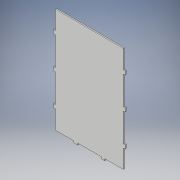
# Autodesk Inventor part: BB Gun Floor
Saved by Autodesk Inventor 2018 (Build 220112000, 112)
## iProperties
Created: 2019-05-24
Part Number: BB Gun Floor
Material: Generic
Document SubType Name: Modeling
Designer: 871357
Density: 1 g/cm^3
Appearance: Default
Author: 871357
Autodesk Inventor part; units mm, degrees
ref_plane "YZ Plane" through (0, 0, 0) normal (1, 0, 0) x (0, 1, 0)
ref_plane "XZ Plane" through (0, 0, 0) normal (0, 1, 0) x (-1, 0, 0)
ref_plane "XY Plane" through (0, 0, 0) normal (0, 0, 1) x (1, 0, 0)
sketch "Sketch1" plane through (0, 0, 0) normal (0, 0, 1) x (1, 0, 0)
  line L0 (0, 0) -> (139.7, 0)
  line L1 (139.7, 0) -> (139.7, 215.9)
  line L2 (139.7, 215.9) -> (0, 215.9)
  line L3 (0, 215.9) -> (0, 0)
  line L4 (38.1, 0) -> (45.72, 0)
  line L5 (45.72, 0) -> (45.72, -3.81)
  line L6 (45.72, -3.81) -> (38.1, -3.81)
  line L7 (38.1, -3.81) -> (38.1, 0)
  line L8 (93.98, 0) -> (101.6, 0)
  line L9 (101.6, 0) -> (101.6, -3.81)
  line L10 (101.6, -3.81) -> (93.98, -3.81)
  line L11 (93.98, -3.81) -> (93.98, 0)
  line L12 (139.7, 38.1) -> (143.51, 38.1)
  line L13 (143.51, 38.1) -> (143.51, 45.72)
  line L14 (143.51, 45.72) -> (139.7, 45.72)
  line L15 (139.7, 45.72) -> (139.7, 38.1)
  line L16 (139.7, 104.14) -> (143.51, 104.14)
  line L17 (143.51, 104.14) -> (143.51, 111.76)
  line L18 (143.51, 111.76) -> (139.7, 111.76)
  line L19 (139.7, 111.76) -> (139.7, 104.14)
  line L20 (139.7, 177.8) -> (143.51, 177.8)
  line L21 (143.51, 177.8) -> (143.51, 170.18)
  line L22 (143.51, 170.18) -> (139.7, 170.18)
  line L23 (139.7, 170.18) -> (139.7, 177.8)
  line L24 (69.85, 215.9) -> (69.85, 61.3437) construction
  line L25 (0, 38.1) -> (-3.81, 38.1)
  line L26 (-3.81, 38.1) -> (-3.81, 45.72)
  line L27 (-3.81, 45.72) -> (0, 45.72)
  line L28 (0, 104.14) -> (-3.81, 104.14)
  line L29 (-3.81, 104.14) -> (-3.81, 111.76)
  line L30 (-3.81, 111.76) -> (0, 111.76)
  line L31 (0, 177.8) -> (-3.81, 177.8)
  line L32 (-3.81, 177.8) -> (-3.81, 170.18)
  line L33 (-3.81, 170.18) -> (0, 170.18)
  line L34 (0, 177.8) -> (0, 170.18)
  line L35 (0, 111.76) -> (0, 104.14)
  line L36 (0, 45.72) -> (0, 38.1)
  line L37 (38.1, 0) -> (45.72, 0)
  line L38 (93.98, 0) -> (101.6, 0)
  dimension "d0" = 139.7
  dimension "d1" = 215.9
  dimension "d2" = 7.62
  dimension "d3" = 3.81
  dimension "d4" = 7.62
  dimension "d5" = 3.81
  dimension "d6" = 38.1
  dimension "d7" = 38.1
  dimension "d8" = 3.81
  dimension "d9" = 7.62
  dimension "d10" = 3.81
  dimension "d11" = 7.62
  dimension "d12" = 3.81
  dimension "d13" = 7.62
  dimension "d14" = 38.1
  dimension "d15" = 38.1
  dimension "d16" = 58.42
  constraints: 78 end point, 12 parallel, 12 symmetric about line, 7 perpendicular, 6 horizontal, 5 point on line, 4 collinear, 1 midpoint, 1 vertical
  measures "d0" distance of L2.end L1.end
  measures "d1" distance of L1.end L0.end
  measures "d2" distance of L5.end L6.end
  measures "d3" distance of L4.end L5.end
  measures "d4" distance of L9.end L10.end
  measures "d5" distance of L8.end L9.end
  measures "d6" distance between parallel lines of L1 L9
  measures "d7" distance between parallel lines of L3 L7
  measures "d8" distance of L14.end L13.end
  measures "d9" distance of L13.end L12.end
  measures "d10" distance of L18.end L17.end
  measures "d11" distance of L17.end L16.end
  measures "d12" distance of L21.end L22.end
  measures "d13" distance of L20.end L21.end
  measures "d14" distance between parallel lines of L2 L20
  measures "d15" distance between parallel lines of L0 L12
  measures "d16" distance from line of L16 L13.end
extrude "Extrusion1" add sketch "Sketch1" along normal blind 2.54
body "Solid1"
